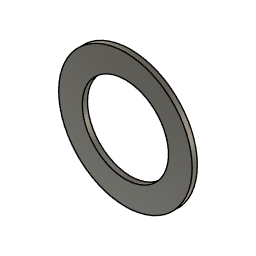
Silicone (Autodesk Fusion 360 design; units mm, degrees)
Autodesk Fusion 360 part; units mm, degrees
sketch "Boceto1" plane through (0, 0, 0) normal (0, 1, 0) x (1, 0, 0)
  circle A0 centre (0, 0) radius 3.5
  circle A1 centre (137.0962, -77.672) radius 22.5 construction
  line L0 (138.2266, -100.1436) -> (138.2266, -104.1436) construction
  circle A2 centre (137.0962, -77.672) radius 26.4957 construction
  circle A3 centre (138.2266, -104.1436) radius 2
  circle A4 centre (156.6138, -95.591) radius 2
  circle A5 centre (163.5678, -76.5416) radius 2
  circle A6 centre (155.0151, -58.1545) radius 2
  circle A7 centre (135.9658, -51.2005) radius 2
  circle A8 centre (117.5787, -59.7531) radius 2
  circle A9 centre (110.6246, -78.8025) radius 2
  circle A10 centre (119.1773, -97.1896) radius 2
  circle A11 centre (138.2266, -104.1436) radius 4.5
  circle A12 centre (156.6138, -95.591) radius 4.5
  circle A13 centre (163.5678, -76.5416) radius 4.5
  circle A14 centre (155.0151, -58.1545) radius 4.5
  circle A15 centre (135.9658, -51.2005) radius 4.5
  circle A16 centre (117.5787, -59.7531) radius 4.5
  circle A17 centre (110.6246, -78.8025) radius 4.5
  circle A18 centre (119.1773, -97.1896) radius 4.5
  circle A19 centre (137.0962, -77.672) radius 21.9957
  circle A20 centre (137.0962, -77.672) radius 30.9957
  circle A21 centre (137.0962, -77.672) radius 21
  circle A22 centre (137.0962, -77.672) radius 32.5
  dimension "d1" = 7
  dimension "d3" = 45
  dimension "d4" = 4
  dimension "d5" = 4
  dimension "d7" = 360
  dimension "d8" = 9
  dimension "d10" = 360
  dimension "d17" = 42
  dimension "d18" = 65
  constraint coincident A0.centre origin
  constraint coincident A1 L0.start
  constraint vertical L0
  constraint concentric A1 A2
  constraint coincident L0.end A2
  constraint coincident L0.end A3.centre
  constraint concentric A3 A11
  constraint concentric A2 A19
  constraint tangent A18 A19
  constraint concentric A19 A20
  constraint tangent A18 A20
  constraint concentric A2 A21
  constraint concentric A2 A22
  measures "d1" diameter of A0
  measures "d3" diameter of A1
  measures "d4" distance of L0.start L0.end
  measures "d5" diameter of A3
  measures "d8" diameter of A11
  measures "d17" diameter of A21
  measures "d18" diameter of A22
extrude "Extruir1" add sketch "Boceto1" along normal blind 2.5 contours A3 | A4 | A5 | A6 | A7 | A8 | A9 | A10 | A19 | A22 makes body 1 at (165.4108, 1.6667, 75.7648) makes body 2 at (108.8682, 1.6667, 77.846) makes body 3 at (119.5762, 1.6667, 59.8528) makes body 4 at (158.4567, 1.6667, 94.8141) makes body 5 at (154.1027, 0.8333, 59.9342) makes body 6 at (117.4209, 1.6667, 96.2331) makes body 7 at (133.2767, 0.8333, 99.3336) makes body 8 at (135.0534, 0.8333, 52.9802) makes body 9 at (140.0696, 1.6667, 103.3668) makes body 10 at (169.5558, 1.6667, 79.292)
extrude "Extruir3" add sketch "Boceto1" 6 faces at (136.3854, 0, 52.3499) (162.5252, 0, 96.9634) (124.4945, 0, 60.1173) (116.698, 0, 60.2359) (111.0403, 0, 78.0825) (119.593, 0, 96.4697) along normal blind 1 contours A3 | A4 | A5 | A6 | A7 | A8 | A9 | A10 | A11 | A11 A12 A19 A20 | A11 A18 A19 A20 | A19 | A18 | A17 A18 A19 A20 | A12 A13 A19 A20 | A12 | A17 | A16 A17 A19 A20 | A16 | A15 A16 A19 A20 | A13 A14 A19 A20 | A13 | A15 | A14 A15 A19 A20 | A14 | A21 | A22 on bodies 2 3 6 7 8 10 bodies 1 8 10 2 3 4 5 6 7 9
delete_face "SuprimirCaras2" 1 faces at (140.5962, 1, 69.5233) on bodies 1
equation "d3 = 80 mm - 35 mm"
equation "d17 = 77 mm - 35 mm"
equation "d18 = 100 mm - 35 mm"
named bodies: "Silicone"
